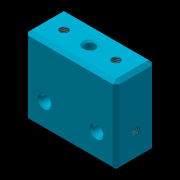
# Autodesk Inventor part: 5190-16-0001
Saved by Autodesk Inventor 2015 (Build 190159000, 159)
## iProperties
Created: 2015-10-17
Part Number: 5190-16-0001
Material: Aluminum 6061
Document SubType Name: Modeling
Designer: JAKE
Mass: 76.7782 g
Surface Area: 81.6796 cm^2
Volume: 28.4364 cm^3
Density: 2.7 g/cm^3
Appearance: Aluminum - Flat
Author: JAKE
Title: ADAPTER BLOCK
Autodesk Inventor part; units mm, degrees
ref_plane "YZ Plane" through (0, 0, 0) normal (1, 0, 0) x (0, 1, 0)
ref_plane "XY Plane" through (0, 0, 0) normal (0, 0, 1) x (1, 0, 0)
sketch "Sketch2" plane through (0, 0, 0) normal (0, 1, 0) x (-1, 0, 0)
  line L0 (0, -13.335) -> (0, 13.335) construction
  line L1 (-31.115, 0) -> (31.115, 0) construction
  line L2 (22.225, 9.525) -> (-22.225, 9.525)
  line L3 (-22.225, 9.525) -> (-22.225, -9.525)
  line L4 (-22.225, -9.525) -> (22.225, -9.525)
  line L5 (22.225, -9.525) -> (22.225, 9.525)
  point P0 (0, 0)
  point P1 (0, 0)
  point P2 (-12.7, 0)
  point P3 (12.7, 0)
  dimension "d0" = 19.05
  dimension "d1" = 44.45
  dimension "d5" = 25.4
  constraints: 8 end point, 2 parallel, 2 point on line, 1 coincident, 1 horizontal, 1 perpendicular, 1 symmetric about line, 2 other
  measures "d0" distance between parallel lines of L4 L2
  measures "d1" distance between parallel lines of L3 L5
  measures "d5" distance of point (-12.7, 0) point (12.7, 0)
extrude "Extrusion1" add sketch "Sketch2" against normal blind 38.1
hole "Hole1" at (0, 0, 0) direction (0, -1, 0) diameter 5.1054 end through all
hole "Hole2" at (12.7, 0, 0) at (-12.7, 0, 0) direction (0, -1, 0) diameter 3.9624 depth 13.6144 tip angle 118 thread size "10-32 UNF" class "2B" standard "ANSI Unified Screw Threads"
ref_plane "Work Plane1" through (0, -25.4, 0) normal (0, 1, 0) x (-1, 0, 0)
sketch "Sketch3" plane through (22.225, 0, -9.525) normal (0, 0, -1) x (-1, 0, 0)
  line L0 (22.225, -45.72) -> (22.225, 7.62) construction
  line L1 (-8.89, -25.4) -> (53.34, -25.4) construction
  line L2 (-8.89, 0) -> (53.34, 0) construction
  point P0 (22.225, 0)
  point P1 (34.925, -25.4)
  point P2 (9.525, -25.4)
  dimension "d21" = 25.4
  constraints: 2 point on line, 1 symmetric about line
  measures "d21" distance of point (9.525, -25.4) point (34.925, -25.4)
hole "Hole3" at (-12.7, -25.4, -9.525) at (12.7, -25.4, -9.525) direction (0, 0, 1) diameter 5.1054 end through all clearance for "Socket Head Cap Screw" size "#10" standard "Ansi Unified Screw Threads"
sketch "Sketch4" plane through (0, -25.4, 0) normal (0, 1, 0) x (-1, 0, 0)
  point P0 (0, 0)
sketch "Sketch5" plane through (-22.225, 0, -9.525) normal (-1, 0, 0) x (0, 0, 1)
  line L0 (9.525, 7.62) -> (9.525, -45.72) construction
  line L1 (-3.81, 0) -> (22.86, 0) construction
  line L2 (-3.81, -25.4) -> (22.86, -25.4) construction
  point P0 (9.525, 0)
  point P1 (9.525, -25.4)
  constraints: 1 midpoint, 1 point on line
hole "Hole4" at (-22.225, -25.4, 0) direction (1, 0, 0) diameter 3.9624 depth 13.6144 tip angle 118 thread size "10-32 UNF" class "2B" standard "ANSI Unified Screw Threads"
mirror "Mirror1" about plane through (0, 0, 0) normal (1, 0, 0) of "Hole4"
chamfer "Chamfer1" distance 1.5875 angle 45 12 edges at (-22.225, -19.05, -9.525) (22.225, -19.05, -9.525) (-22.225, -19.05, 9.525) (22.225, -19.05, 9.525) (0, 0, 9.525) (0, 0, -9.525) (-22.225, 0, 0) (22.225, 0, 0) (0, -38.1, 9.525) (22.225, -38.1, 0) (0, -38.1, -9.525) (-22.225, -38.1, 0)
chamfer "Chamfer2" distance 0.7937 angle 45 6 edges at (-12.7, -27.9527, 9.525) (12.7, -27.9527, 9.525) (12.7, -27.9527, -9.525) (-12.7, -27.9527, -9.525) (0, 0, -2.5527) (0, -38.1, -2.5527)
equation "\"d21\" = d5"
body "Solid1"
